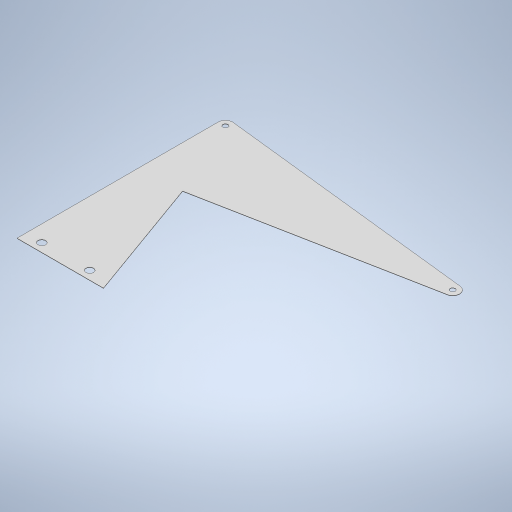
# Autodesk Inventor part: base_main_pcb_p1
Saved by Autodesk Inventor 2024 (Build 280153000, 153)
## iProperties
Created: 2026-03-21
Part Number: base_main_pcb_p1
Material: Generic
Document SubType Name: Modeling
Designer: schar
Density: 1 g/cm^3
Appearance: Default
Author: schar
Autodesk Inventor part; units mm, degrees
ref_plane "YZ Plane" through (0, 0, 0) normal (1, 0, 0) x (0, 1, 0)
ref_plane "XZ Plane" through (0, 0, 0) normal (0, 1, 0) x (-1, 0, 0)
ref_plane "Work Plane1" through (-197.5, 0.2, 285.96) normal (0, -1, 0) x (1, 0, 0)
sketch "Sketch1" plane through (-197.5, 0.2, 285.96) normal (0, -1, 0) x (1, 0, 0)
  line L0 (51.2973, -136.9464) -> (22.584, -216.7184) projected
  line L1 (51.2973, -136.9464) -> (-4.5, -136.9464)
  line L2 (-4.5, -266.96) -> (-4.5, -4.5) projected
  line L3 (51.2973, -136.9464) -> (22.584, -216.7184)
  line L4 (22.584, -216.7184) -> (165, -244.16) projected
  line L5 (22.584, -216.7184) -> (165, -244.16)
  circle A0 centre (165, -248.66) radius 1.675 projected
  circle A1 centre (165, -248.66) radius 4.5
  arc A2 (-4.5, -266.96) -> (0.561, -271.4249) centre (0, -266.96) ccw projected
  line L6 (165, -253.16) -> (0.561, -271.4249) projected
  circle A3 centre (0, -266.96) radius 4.5
  line L7 (-4.5, -266.96) -> (-4.5, -136.9464)
  circle A4 centre (165, -248.66) radius 1.675
  circle A5 centre (0, -266.96) radius 1.675
  circle A6 centre (36.9406, -142.4458) radius 2.5 projected
  circle A7 centre (36.9406, -142.4458) radius 2.5
  circle A8 centre (5.9848, -142.4458) radius 2.5 projected
  circle A9 centre (5.9848, -142.4458) radius 2.5
  line L8 (165, -253.16) -> (0, -271.46)
  point P0 (197.5, -285.96)
  constraints: 10 end point, 6 centre point, 6 coincident, 3 point on circle, 1 collinear, 1 concentric, 1 horizontal, 1 perpendicular, 1 point on line
extrude "Extrusion1" add sketch "Sketch1" along normal blind 0.2 contours L0 L4 A1 L8 A3 L2 L1 | A1 | A3 L8 A2 picked at (-3.4985, -266.4674)
body "Solid2"
